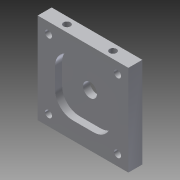
# Autodesk Inventor part: motor_mount
Saved by Autodesk Inventor 2013 (Build 170138000, 138)
## iProperties
Created: 2013-07-22
Part Number: motor_mount
Material: Generic
Document SubType Name: Modeling
Designer: pnyholm
Density: 1 g/cm^3
Author: pnyholm
Autodesk Inventor part; units mm, degrees
ref_plane "YZ Plane" through (0, 0, 0) normal (1, 0, 0) x (0, 1, 0)
ref_plane "XZ Plane" through (0, 0, 0) normal (0, 1, 0) x (-1, 0, 0)
ref_plane "XY Plane" through (0, 0, 0) normal (0, 0, 1) x (1, 0, 0)
sketch "Sketch1" plane through (0, 0, 0) normal (0, 0, 1) x (1, 0, 0)
  line L0 (0, 0) -> (41.275, 0)
  line L1 (41.275, 0) -> (41.275, 41.275)
  line L2 (41.275, 41.275) -> (0, 41.275)
  line L3 (0, 41.275) -> (0, 0)
  circle A0 centre (20.6375, 20.6375) radius 22.225 construction
  line L4 (0, 0) -> (41.275, 41.275) construction
  line L5 (0, 41.275) -> (41.275, 0) construction
  circle A1 centre (4.9221, 36.3529) radius 1.5875
  circle A2 centre (4.9221, 4.9221) radius 1.5875
  circle A3 centre (36.3529, 36.3529) radius 1.5875
  circle A4 centre (36.3529, 4.9221) radius 1.5875
  dimension "d0" = 41.275
  dimension "d2" = 41.275
  dimension "d3" = 44.45
  dimension "d4" = 3.175
  dimension "d5" = 3.175
  dimension "d6" = 3.175
  dimension "d7" = 3.175
  dimension "d8" = 20.6375
  dimension "d9" = 20.6375
  constraints: 12 end point, 5 centre point, 4 point on circle, 4 point on line, 2 parallel, 1 horizontal, 1 perpendicular
  measures "d0" distance of L0.end L1.end
  measures "d2" distance of L1.end L2.end
  measures "d3" diameter of A0
  measures "d4" diameter of A1
  measures "d5" diameter of A2
  measures "d6" diameter of A3
  measures "d7" diameter of A4
  measures "d8" distance from line of A0.centre L1
  measures "d9" distance from line of A0.centre L0
extrude "Extrusion1" add sketch "Sketch1" along normal blind 6.35
sketch "Sketch2" plane through (0, 41.275, 0) normal (0, 1, 0) x (1, 0, 0)
  line L0 (41.275, 0) -> (0, 0) projected
  line L1 (0, 0) -> (0, -6.35) projected
  line L2 (41.275, 0) -> (41.275, -6.35) projected
  circle A0 centre (10.16, -3.175) radius 1.5964
  circle A1 centre (31.115, -3.175) radius 1.5964
  dimension "d12" = 3.1928
  dimension "d14" = 3.1928
  dimension "d15" = 10.16
  dimension "d17" = 10.16
  dimension "d18" = 3.175
  dimension "d19" = 3.175
  constraints: 2 centre point
  measures "d12" diameter of A0
  measures "d14" diameter of A1
  measures "d15" distance from line of L1 A0.centre
  measures "d17" distance from line of A1.centre L2
  measures "d18" distance from line of L0 A0.centre
  measures "d19" distance from line of L0 A1.centre
extrude "Extrusion2" cut sketch "Sketch2" against normal blind 6.35
sketch "Sketch3" plane through (0, 0, 6.35) normal (0, 0, 1) x (1, 0, 0)
  line L0 (7.9375, 7.9375) -> (33.3375, 7.9375)
  line L1 (33.3375, 7.9375) -> (33.3375, 33.3375)
  line L2 (33.3375, 33.3375) -> (7.9375, 33.3375)
  line L3 (7.9375, 33.3375) -> (7.9375, 7.9375)
  constraints: 8 end point, 2 parallel, 1 horizontal, 1 perpendicular
extrude "Extrusion3" cut sketch "Sketch3" against normal blind 3.175
fillet "Fillet1" radius 7.9375 1 edges at (7.9375, 33.3375, 4.7625)
fillet "Fillet2" radius 7.9375 3 edges at (7.9375, 7.9375, 4.7625) (33.3375, 7.9375, 4.7625) (33.3375, 33.3375, 4.7625)
sketch "Sketch4" plane through (0, 0, 3.175) normal (0, 0, 1) x (1, 0, 0)
  circle A0 centre (20.6375, 20.6375) radius 3.175
  point P0 (0, 0)
  dimension "d33" = 6.35
  constraints: 1 centre point
  measures "d33" diameter of A0
extrude "Extrusion4" cut sketch "Sketch4" against normal blind 25.4
body "Solid1"
